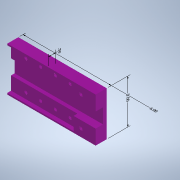
# Autodesk Inventor part: pistonHousing
Saved by Autodesk Inventor 2020.2 (Build 242310000, 310)
## iProperties
Created: 2020-01-13
Part Number: pistonHousing
Material: PET Plastic
Document SubType Name: Modeling
Designer: robst
Density: 1.541 g/cm^3
Appearance: Smooth - Purple
Author: robst
Autodesk Inventor part; units mm, degrees
ref_plane "YZ Plane" through (0, 0, 0) normal (1, 0, 0) x (0, 1, 0)
ref_plane "XZ Plane" through (0, 0, 0) normal (0, 1, 0) x (-1, 0, 0)
ref_plane "XY Plane" through (0, 0, 0) normal (0, 0, 1) x (1, 0, 0)
sketch "Sketch1" plane through (0, 0, 0) normal (0, 0, 1) x (1, 0, 0)
  line L0 (-76.2, -38.1) -> (76.2, -38.1)
  line L1 (76.2, -38.1) -> (76.2, 38.1)
  line L2 (76.2, 38.1) -> (-76.2, 38.1)
  line L3 (-76.2, 38.1) -> (-76.2, -38.1)
  line L4 (-76.2, -38.1) -> (76.2, 38.1) construction
  line L5 (76.2, -38.1) -> (-76.2, 38.1) construction
  point P0 (0, 0)
  dimension "d0" = 152.4
  dimension "d1" = 76.2
  constraints: 12 end point, 2 midpoint, 2 parallel, 1 horizontal, 1 perpendicular
  measures "d0" distance of L2.end L1.end
  measures "d1" distance of L1.end L0.end
extrude "Extrusion1" add sketch "Sketch1" along normal mid plane 19.05
sketch "Sketch3" plane through (0, 0, 9.525) normal (0, 0, 1) x (1, 0, 0)
  line L0 (-76.2, -12.7) -> (76.2, -12.7)
  line L1 (76.2, -12.7) -> (76.2, 12.7)
  line L2 (76.2, 12.7) -> (-76.2, 12.7)
  line L3 (-76.2, 12.7) -> (-76.2, -12.7)
  line L4 (-76.2, -12.7) -> (76.2, 12.7) construction
  line L5 (76.2, -12.7) -> (-76.2, 12.7) construction
  point P0 (0, 0)
  dimension "d7" = 25.4
  dimension "d19" = 152.4
  constraints: 12 end point, 2 midpoint, 2 parallel, 1 horizontal, 1 perpendicular
  measures "d7" distance of L1.end L0.end
  measures "d19" distance of L1.end L2.end
extrude "Extrusion3" cut sketch "Sketch3" against normal blind 12.7
ref_plane "Work Plane1" through (-76.2, 38.1, 9.525) normal (0, 0, 1) x (1, 0, 0)
sketch "Sketch4" plane through (0, 0, 9.525) normal (0, 0, 1) x (1, 0, 0)
  line L0 (-76.2, 38.1) -> (-76.2, 12.7) construction
  line L1 (-76.2, 25.4) -> (76.2, 25.4) construction
  line L2 (76.2, 38.1) -> (76.2, -38.1) construction
  line L3 (-76.2, -12.7) -> (-76.2, 12.7) construction
  line L4 (-76.2, 0) -> (76.2, 0) construction
  point P0 (0, 0)
  point P1 (-50.8, 25.4)
  point P2 (-25.4, 25.4)
  point P3 (0, 25.4)
  point P4 (25.4, 25.4)
  point P5 (50.8, 25.4)
  point P6 (-50.8, -25.4)
  point P7 (-25.4, -25.4)
  point P8 (0, -25.4)
  point P9 (25.4, -25.4)
  point P10 (50.8, -25.4)
  dimension "d20" = 25.4
  dimension "d23" = 25.4
  constraints: 5 symmetric about line, 4 end point, 3 midpoint, 2 horizontal, 2 point on line, 4 other
  measures "d20" distance from line of point (-50.8, 25.4) L0
  measures "d23" distance of point (-50.8, 25.4) point (-25.4, 25.4)
hole "Hole1" at (-50.8, 25.4, 9.525) at (-25.4, 25.4, 9.525) at (0, 25.4, 9.525) at (25.4, 25.4, 9.525) at (50.8, 25.4, 9.525) at (-50.8, -25.4, 9.525) at (-25.4, -25.4, 9.525) at (0, -25.4, 9.525) at (25.4, -25.4, 9.525) at (50.8, -25.4, 9.525) direction (0, 0, -1) diameter 5.1054 end through all clearance for "Hex Machine Screw" size "#10" standard "Ansi Unified Screw Threads"
sketch "Sketch6" plane through (0, 0, 9.525) normal (0, 0, 1) x (1, 0, 0)
  line L0 (-76.2, -35.56) -> (38.1, -35.56)
  line L1 (38.1, -35.56) -> (38.1, 35.56)
  line L2 (38.1, 35.56) -> (-76.2, 35.56)
  line L3 (-76.2, 35.56) -> (-76.2, -35.56)
  line L4 (-76.2, -38.1) -> (76.2, -38.1) projected
  line L5 (76.2, 38.1) -> (-76.2, 38.1) projected
  line L6 (76.2, 12.7) -> (76.2, 38.1) projected
  point P0 (0, 0)
  dimension "d40" = 2.54
  dimension "d41" = 2.54
  dimension "d42" = 38.1
  constraints: 8 end point, 2 parallel, 1 horizontal, 1 perpendicular
  measures "d40" distance between parallel lines of L4 L0
  measures "d41" distance between parallel lines of L2 L5
  measures "d42" distance between parallel lines of L6 L1
extrude "Extrusion4" cut sketch "Sketch6" against normal blind 6.604
body "Solid1"
